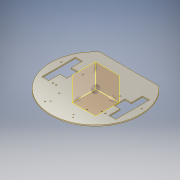
# Autodesk Inventor part: BottomPlate
Saved by Autodesk Inventor 2019 (Build 230136000, 136)
## iProperties
Created: 2020-02-28
Part Number: BottomPlate
Material: Generic
Document SubType Name: Modeling
Designer: james
Mass: 617.778 g
Surface Area: 2655.15 cm^2
Volume: 617.778 cm^3
Density: 1 g/cm^3
Appearance: Titanium
Author: james
Autodesk Inventor part; units mm, degrees
ref_plane "YZ Plane" through (0, 0, 0) normal (1, 0, 0) x (0, 1, 0)
ref_plane "XZ Plane" through (0, 0, 0) normal (0, 1, 0) x (-1, 0, 0)
ref_plane "XY Plane" through (0, 0, 0) normal (0, 0, 1) x (1, 0, 0)
sketch "Sketch1" plane through (0, 0, 0) normal (0, 1, 0) x (-1, 0, 0)
  circle A0 centre (0, 0) radius 203.2
  dimension "d0" = 406.4
  constraints: 1 centre point, 1 coincident
  measures "d0" diameter of A0
extrude "Extrusion1" add sketch "Sketch1" along normal blind 4.7625
sketch "Sketch2" plane through (0, 4.7625, 0) normal (0, 1, 0) x (1, 0, 0)
  line L0 (-165.1, -76.2) -> (-139.7, -76.2)
  line L1 (-139.7, -76.2) -> (-139.7, 76.2)
  line L2 (-139.7, 76.2) -> (-165.1, 76.2)
  line L3 (-165.1, 76.2) -> (-165.1, -76.2)
  line L4 (139.7, 76.2) -> (165.1, 76.2)
  line L5 (165.1, 76.2) -> (165.1, -76.2)
  line L6 (165.1, -76.2) -> (139.7, -76.2)
  line L7 (139.7, -76.2) -> (139.7, 76.2)
  point P0 (0, 0)
  dimension "d3" = 25.4
  dimension "d4" = 25.4
  dimension "d5" = 0
  dimension "d6" = 0
  dimension "d7" = 152.4
  dimension "d8" = 76.2
  dimension "d9" = 139.7
  dimension "d10" = 139.7
  constraints: 16 end point, 4 parallel, 2 horizontal, 2 perpendicular
  measures "d3" distance of L5.end L6.end
  measures "d4" distance of L0.start L0.end
  measures "d5" distance between parallel lines of L6 L0
  measures "d6" distance between parallel lines of L4 L2
  measures "d7" distance of L4.end L5.end
  measures "d8" distance from line of point (0, 0) L6
  measures "d9" distance from line of L1 point (0, 0)
  measures "d10" distance from line of L7 point (0, 0)
extrude "Extrusion2" cut sketch "Sketch2" against normal blind 28.575
sketch "Sketch4" plane through (0, 0, 0) normal (0, -1, 0) x (1, 0, 0)
  line L0 (-136.525, 76.2) -> (-167.64, 76.2)
  line L1 (-167.64, 76.2) -> (-167.64, -76.2)
  line L2 (-167.64, -76.2) -> (-136.525, -76.2)
  line L3 (-136.525, -76.2) -> (-136.525, 76.2)
  line L4 (-139.7, -76.2) -> (-165.1, -76.2) projected
  line L5 (-165.1, 76.2) -> (-139.7, 76.2) projected
  line L6 (-165.1, -76.2) -> (-165.1, 76.2) projected
  line L7 (-139.7, 76.2) -> (-139.7, -76.2) projected
  point P0 (0, 0)
  dimension "d24" = 0
  dimension "d25" = 0
  dimension "d26" = 2.54
  dimension "d27" = 3.175
  constraints: 8 end point, 2 parallel, 1 horizontal, 1 perpendicular
  measures "d24" distance between parallel lines of L2 L4
  measures "d25" distance between parallel lines of L5 L0
  measures "d26" distance between parallel lines of L6 L1
  measures "d27" distance between parallel lines of L7 L3
extrude "Extrusion3" cut sketch "Sketch4" against normal blind 11.1125 contours L3 L2 L7 L0 | L6 L2 L1 L0
sketch "Sketch6" plane through (0, 0, 0) normal (0, -1, 0) x (1, 0, 0)
  point P0 (0, 0)
  point P1 (52.197, 152.4)
  point P2 (-52.197, 152.4)
  dimension "d48" = 0
  dimension "d49" = 104.394
  dimension "d50" = 52.197
  dimension "d51" = 152.4
  measures "d48" vertical distance of point (-52.197, 152.4) point (52.197, 152.4)
  measures "d49" distance of point (-52.197, 152.4) point (52.197, 152.4)
  measures "d50" horizontal distance of point (0, 0) point (52.197, 152.4)
  measures "d51" vertical distance of point (0, 0) point (-52.197, 152.4)
hole "Hole3" at (52.197, 0, 152.4) at (-52.197, 0, 152.4) direction (0, 1, 0) diameter 3.81 depth 25.4 tip angle 118
sketch "Sketch8" plane through (0, 4.7625, 0) normal (0, 1, 0) x (1, 0, 0)
  line L0 (-249.9736, 258.2829) -> (238.9858, 258.2829)
  line L1 (238.9858, 258.2829) -> (238.9858, 152.4)
  line L2 (238.9858, 152.4) -> (-249.9736, 152.4)
  line L3 (-249.9736, 152.4) -> (-249.9736, 258.2829)
  point P0 (0, 0)
  dimension "d80" = 152.4
  constraints: 8 end point, 2 parallel, 1 horizontal, 1 perpendicular
  measures "d80" distance from line of point (0, 0) L2
extrude "Extrusion4" cut sketch "Sketch8" against normal blind 100.0125
sketch "Sketch9" plane through (0, 4.7625, 0) normal (0, 1, 0) x (1, 0, 0)
  line L0 (-142.7514, 25.4) -> (-104.775, 25.4)
  line L1 (-104.775, 25.4) -> (-104.775, -25.4)
  line L2 (-104.775, -25.4) -> (-142.7514, -25.4)
  line L3 (-142.7514, -25.4) -> (-142.7514, 25.4)
  line L4 (-136.525, 76.2) -> (-136.525, -76.2) projected
  line L5 (-167.64, 76.2) -> (-136.525, 76.2) projected
  point P0 (0, 0)
  dimension "d83" = 50.8
  dimension "d84" = 31.75
  dimension "d85" = 50.8
  constraints: 8 end point, 2 parallel, 1 horizontal, 1 perpendicular
  measures "d83" distance of L0.end L1.end
  measures "d84" distance between parallel lines of L4 L1
  measures "d85" distance between parallel lines of L5 L0
extrude "Extrusion5" cut sketch "Sketch9" against normal blind 9.525
sketch "Sketch10" plane through (0, 4.7625, 0) normal (0, 1, 0) x (1, 0, 0)
  line L0 (149.2619, 25.4) -> (107.95, 25.4)
  line L1 (107.95, 25.4) -> (107.95, -25.4)
  line L2 (107.95, -25.4) -> (149.2619, -25.4)
  line L3 (149.2619, -25.4) -> (149.2619, 25.4)
  line L4 (-104.775, -25.4) -> (-136.525, -25.4) projected
  line L5 (-136.525, 25.4) -> (-104.775, 25.4) projected
  line L6 (139.7, -76.2) -> (139.7, 76.2) projected
  point P0 (0, 0)
  dimension "d97" = 0
  dimension "d98" = 0
  dimension "d99" = 31.75
  constraints: 8 end point, 2 parallel, 1 horizontal, 1 perpendicular
  measures "d97" distance between parallel lines of L4 L2
  measures "d98" distance between parallel lines of L5 L0
  measures "d99" distance between parallel lines of L1 L6
extrude "Extrusion6" cut sketch "Sketch10" against normal blind 25.4
sketch "Sketch11" plane through (0, 4.7625, 0) normal (0, 1, 0) x (1, 0, 0)
  line L0 (-136.525, -76.2) -> (-167.64, -76.2) projected
  line L1 (-136.525, -25.4) -> (-136.525, -76.2) projected
  line L2 (139.7, -76.2) -> (139.7, -25.4) projected
  point P0 (0, 0)
  point P1 (-117.475, -76.2)
  point P2 (-102.235, -76.2)
  point P3 (105.41, -76.2)
  point P4 (120.65, -76.2)
  dimension "d102" = 0
  dimension "d103" = 0
  dimension "d104" = 0
  dimension "d105" = 0
  dimension "d106" = 15.24
  dimension "d107" = 15.24
  dimension "d108" = 19.05
  dimension "d109" = 19.05
  measures "d102" vertical distance of point (105.41, -76.2) point (120.65, -76.2)
  measures "d103" vertical distance of point (-102.235, -76.2) point (105.41, -76.2)
  measures "d104" vertical distance of point (-102.235, -76.2) point (-117.475, -76.2)
  measures "d105" distance from line of L0 point (-117.475, -76.2)
  measures "d106" distance of point (-102.235, -76.2) point (-117.475, -76.2)
  measures "d107" distance of point (120.65, -76.2) point (105.41, -76.2)
  measures "d108" distance from line of point (-117.475, -76.2) L1
  measures "d109" distance from line of L2 point (120.65, -76.2)
hole "Hole5" at (-117.475, 4.7625, 76.2) at (-102.235, 4.7625, 76.2) at (105.41, 4.7625, 76.2) at (120.65, 4.7625, 76.2) direction (0, -1, 0) diameter 5.1054 depth 25.4 tip angle 118 clearance for "Hex Machine Screw" size "#10" standard "Ansi Unified Screw Threads"
sketch "Sketch12" plane through (0, 4.7625, 0) normal (0, 1, 0) x (1, 0, 0)
  circle A0 centre (105.41, -76.2) radius 2.5527 projected
  circle A1 centre (-102.235, -76.2) radius 2.5527 projected
  point P0 (0, 0)
  point P1 (-83.185, 25.4)
  point P2 (86.36, 25.4)
  point P3 (-180.975, 25.4)
  point P4 (184.15, 25.4)
  dimension "d117" = 101.6
  dimension "d118" = 19.05
  dimension "d119" = 19.05
  dimension "d120" = 101.6
  dimension "d121" = 0
  dimension "d122" = 0
  dimension "d123" = 97.79
  dimension "d124" = 97.79
  measures "d117" vertical distance of A1.centre point (-83.185, 25.4)
  measures "d118" horizontal distance of A1.centre point (-83.185, 25.4)
  measures "d119" horizontal distance of A0.centre point (86.36, 25.4)
  measures "d120" vertical distance of A0.centre point (86.36, 25.4)
  measures "d121" vertical distance of point (184.15, 25.4) point (86.36, 25.4)
  measures "d122" vertical distance of point (-83.185, 25.4) point (-180.975, 25.4)
  measures "d123" distance of point (-83.185, 25.4) point (-180.975, 25.4)
  measures "d124" distance of point (86.36, 25.4) point (184.15, 25.4)
hole "Hole6" at (-83.185, 4.7625, -25.4) at (86.36, 4.7625, -25.4) at (-180.975, 4.7625, -25.4) at (184.15, 4.7625, -25.4) direction (0, -1, 0) diameter 5.1054 depth 25.4 tip angle 118 clearance for "Hex Machine Screw" size "#10" standard "Ansi Unified Screw Threads"
sketch "Sketch13" plane through (0, 4.7625, 0) normal (0, 1, 0) x (1, 0, 0)
  line L0 (136.525, -76.2) -> (167.64, -76.2)
  line L1 (167.64, -76.2) -> (167.64, 76.2)
  line L2 (167.64, 76.2) -> (136.525, 76.2)
  line L3 (136.525, 76.2) -> (136.525, -76.2)
  line L4 (139.7, 76.2) -> (165.1, 76.2) projected
  line L5 (165.1, -76.2) -> (139.7, -76.2) projected
  line L6 (139.7, -76.2) -> (139.7, -25.4) projected
  line L7 (165.1, 76.2) -> (165.1, -76.2) projected
  point P0 (0, 0)
  dimension "d132" = 0
  dimension "d133" = 0
  dimension "d134" = 3.175
  dimension "d135" = 2.54
  constraints: 8 end point, 2 parallel, 1 horizontal, 1 perpendicular
  measures "d132" distance between parallel lines of L4 L2
  measures "d133" distance between parallel lines of L5 L0
  measures "d134" distance between parallel lines of L6 L3
  measures "d135" distance between parallel lines of L7 L1
extrude "Extrusion7" cut sketch "Sketch13" against normal blind 14.2875
sketch "Sketch14" plane through (0, 4.7625, 0) normal (0, 1, 0) x (1, 0, 0)
  point P0 (0, 0)
  point P1 (-63.5, -101.6)
  point P2 (63.5, -101.6)
  point P3 (63.5, -165.1)
  point P4 (-63.5, -165.1)
  dimension "d138" = 0
  dimension "d139" = 0
  dimension "d140" = 0
  dimension "d141" = 0
  dimension "d142" = 63.5
  dimension "d143" = 127
  dimension "d144" = 63.5
  dimension "d145" = 101.6
  measures "d138" vertical distance of point (63.5, -101.6) point (-63.5, -101.6)
  measures "d139" vertical distance of point (63.5, -165.1) point (-63.5, -165.1)
  measures "d140" horizontal distance of point (63.5, -101.6) point (63.5, -165.1)
  measures "d141" horizontal distance of point (-63.5, -101.6) point (-63.5, -165.1)
  measures "d142" distance of point (-63.5, -165.1) point (-63.5, -101.6)
  measures "d143" distance of point (63.5, -165.1) point (-63.5, -165.1)
  measures "d144" horizontal distance of point (0, 0) point (63.5, -165.1)
  measures "d145" vertical distance of point (-63.5, -101.6) point (0, 0)
hole "Hole7" at (-63.5, 4.7625, 101.6) at (63.5, 4.7625, 101.6) at (63.5, 4.7625, 165.1) at (-63.5, 4.7625, 165.1) direction (0, -1, 0) diameter 4.4958 depth 25.4 tip angle 118 clearance for "Hex Machine Screw" size "#8" standard "Ansi Unified Screw Threads"
body "Solid1"
